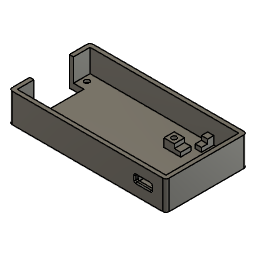
case_body (Autodesk Fusion 360 design; units mm, degrees)
Autodesk Fusion 360 part; units mm, degrees
sketch "Sketch1" plane through (0, 0, 0) normal (0, 1, 0) x (1, 0, 0)
  line L0 (0, 0) -> (75.7, 0)
  line L1 (75.7, 0) -> (75.7, -39.1)
  line L2 (75.7, -39.1) -> (0, -39.1)
  line L3 (0, 0) -> (0, -10)
  line L4 (0, -10) -> (7, -10)
  line L5 (7, -10) -> (7, -29.1)
  line L6 (7, -29.1) -> (0, -29.1)
  line L7 (0, -29.1) -> (0, -39.1)
  dimension "d1" = 75.7
  dimension "d2" = 39.1
  dimension "d67" = 10
  dimension "d68" = 10
  dimension "d69" = 7
  constraint horizontal L0
  constraint vertical L1
  constraint horizontal L2
  constraint coincident L0.start L3.start
  constraint vertical L3
  constraint perpendicular L3 L4
  constraint perpendicular L4 L5
  constraint perpendicular L3 L6
  constraint perpendicular L2 L7
  constraint collinear L3 L7
  measures "d1" distance of L0.start L0.end
  measures "d2" distance of L0.start L2.end
  measures "d67" distance of L0.start L3.end
  measures "d68" distance of L2.end L6.end
  measures "d69" distance of L5.end L6.end
extrude "Extrude1" add sketch "Sketch1" along normal blind 3 makes body 1
sketch "Sketch2" plane through (0, 3, 0) normal (0, 1, 0) x (-1, 0, 0)
  line L0 (-75.7, 0) -> (0, 0)
  line L1 (0, 0) -> (-75.7, 0)
  line L2 (-73.7, 2) -> (-2, 2)
  line L3 (-2, 2) -> (-2, 37.1)
  line L4 (-2, 37.1) -> (-73.7, 37.1)
  line L5 (-73.7, 37.1) -> (-73.7, 2)
  line L6 (0, 39.1) -> (-75.7, 39.1)
  line L7 (0, 0) -> (0, 39.1)
  line L8 (-75.7, 0) -> (-75.7, 39.1)
  line L9 (0, 0) -> (0, 10)
  line L10 (0, 10) -> (-7, 10)
  line L11 (-7, 10) -> (-7, 29.1)
  line L12 (-7, 29.1) -> (0, 29.1)
  line L13 (0, 29.1) -> (0, 39.1)
  point P0 (-75.7, 39.1)
  dimension "d31" = 2
  dimension "d34" = 2
  dimension "d35" = 2
  dimension "d36" = 2
  constraint horizontal L1
  constraint horizontal L2
  constraint coincident L0.end L1.start
  constraint vertical L3
  constraint horizontal L4
  constraint vertical L5
  constraint perpendicular L6 L7
  constraint perpendicular L6 L8
  constraint coincident P0 L6.end
  measures "d31" distance of L1 L2
  measures "d34" distance of L4 L6
  measures "d35" distance of L3 L7
  measures "d36" distance of L5 L8
extrude "Extrude2" add sketch "Sketch2" along normal blind 11 contours L0 L1 L2 L3 L4 L5 L6 L7 L8 L9 L10 L12 L13 bodies 1
sketch "Sketch3" plane through (0, 3, 0) normal (0, 1, 0) x (-1, 0, 0)
  line L0 (-73.7, 2) -> (-70.7, 2)
  line L1 (-70.7, 2) -> (-70.7, 5)
  line L2 (-70.7, 5) -> (-73.7, 5)
  line L3 (-73.7, 5) -> (-73.7, 2)
  line L4 (-55.6, 37.1) -> (-50.6, 37.1)
  line L5 (-50.6, 37.1) -> (-50.6, 32.1)
  line L6 (-50.6, 32.1) -> (-55.6, 32.1)
  line L7 (-55.6, 32.1) -> (-55.6, 37.1)
  line L8 (-58.7, 2) -> (-61.7, 2)
  line L9 (-61.7, 2) -> (-61.7, 5)
  line L10 (-61.7, 5) -> (-58.7, 5)
  line L11 (-58.7, 5) -> (-58.7, 2)
  line L12 (-50.6, 15) -> (-55.6, 15)
  line L13 (-55.6, 15) -> (-55.6, 10)
  line L14 (-50.6, 15) -> (-50.6, 10)
  line L15 (-50.6, 10) -> (-55.6, 10)
  line L16 (-73.7, 2) -> (-73.7, 37.1)
  line L17 (-2, 2) -> (-73.7, 2)
  line L18 (-73.7, 37.1) -> (-2, 37.1)
  dimension "d20" = 5
  dimension "d21" = 5
  dimension "d28" = 3
  dimension "d29" = 5
  dimension "d47" = 3
  dimension "d49" = 5
  dimension "d83" = 3
  dimension "d84" = 12
  dimension "d85" = 18.1
  dimension "d86" = 8
  constraint horizontal L0
  constraint vertical L1
  constraint vertical L3
  constraint horizontal L4
  constraint vertical L5
  constraint horizontal L6
  constraint vertical L7
  constraint horizontal L8
  constraint vertical L9
  constraint vertical L11
  constraint horizontal L12
  constraint vertical L13
  constraint collinear L2 L10
  constraint collinear L7 L13
  constraint perpendicular L9 L10
  constraint perpendicular L12 L14
  constraint coincident L8.start L17
  constraint coincident L0.end L17
  constraint coincident L2.end L16
  constraint coincident L4.end L18
  measures "d20" distance of L5.end L6.end
  measures "d21" distance of L4.end L5.end
  measures "d28" distance of L8.start L8.end
  measures "d29" distance of L12.start L12.end
  measures "d47" horizontal distance of L1.end L2.end
  measures "d49" distance of L12.start L14.end
  measures "d83" distance of L8.start L10.end
  measures "d84" distance of L9 L16
  measures "d85" distance of L7 L16
  measures "d86" distance of L15 L17
extrude "Extrude5" add sketch "Sketch3" along normal blind 4 separate body makes body 2 at (73.7, 4.3333, 4) makes body 3 at (58.7, 4.3333, 4) makes body 4 at (53.9333, 3, 35.4333) makes body 5 at (53.9333, 3, 11.6667)
sketch "Sketch5" plane through (0, 3, 0) normal (0, 1, 0) x (-1, 0, 0)
  line L0 (-70.7, 5) -> (-73.7, 5)
  line L1 (-73.7, 5) -> (-73.7, 8)
  line L2 (-73.7, 8) -> (-70.7, 8)
  line L3 (-70.7, 8) -> (-70.7, 5)
  line L4 (-55.6, 32.1) -> (-58.7, 32.1)
  line L5 (-58.7, 32.1) -> (-58.7, 37.1)
  line L6 (-58.7, 37.1) -> (-55.6, 37.1)
  line L7 (-55.6, 37.1) -> (-55.6, 32.1)
  line L8 (-73.7, 37.1) -> (-70.7, 37.1)
  line L9 (-70.7, 37.1) -> (-70.7, 32.1)
  line L10 (-70.7, 32.1) -> (-73.7, 32.1)
  line L11 (-73.7, 32.1) -> (-73.7, 37.1)
  line L12 (-58.7, 5) -> (-61.7, 5)
  line L13 (-61.7, 5) -> (-61.7, 8)
  line L14 (-61.7, 8) -> (-58.7, 8)
  line L15 (-58.7, 8) -> (-58.7, 5)
  line L16 (-58.7, 10) -> (-58.7, 15)
  line L17 (-58.7, 15) -> (-55.6, 15)
  line L18 (-55.6, 15) -> (-55.6, 10)
  line L19 (-55.6, 10) -> (-58.7, 10)
  line L20 (-2, 29.1) -> (-2, 37.1)
  line L21 (-2, 37.1) -> (-73.7, 37.1)
  line L22 (-73.7, 37.1) -> (-73.7, 2)
  line L23 (-73.7, 2) -> (-2, 2)
  line L24 (-2, 2) -> (-2, 10)
  line L25 (-2, 10) -> (-7, 10)
  line L26 (-7, 10) -> (-7, 29.1)
  line L27 (-7, 29.1) -> (-2, 29.1)
  point P0 (-73.7, 5)
  point P1 (-55.6, 37.1)
  point P2 (-58.7, 5)
  point P3 (-73.7, 37.1)
  point P4 (-55.6, 10)
  point P5 (-55.6, 15)
  point P6 (-61.7, 5)
  point P7 (-70.7, 5)
  point P8 (-55.6, 32.1)
  dimension "d43" = 3
  constraint horizontal L0
  constraint vertical L1
  constraint vertical L3
  constraint coincident P0 L0.end
  constraint horizontal L4
  constraint horizontal L6
  constraint vertical L7
  constraint coincident P1 L6.end
  constraint horizontal L8
  constraint vertical L9
  constraint horizontal L10
  constraint vertical L11
  constraint collinear L3 L9
  constraint collinear L4 L10
  constraint horizontal L12
  constraint vertical L13
  constraint horizontal L14
  constraint vertical L15
  constraint coincident P2 L12.start
  constraint collinear L2 L14
  constraint vertical L16
  constraint horizontal L17
  constraint vertical L18
  constraint collinear L15 L16
  constraint collinear L5 L16
  constraint coincident P3 L8.start
  constraint coincident P4 L18.end
  constraint perpendicular L16 L19
  constraint coincident P5 L17.end
  constraint coincident P6 L12.end
  constraint coincident P7 L0.start
  constraint coincident P8 L4.start
  measures "d43" distance of P2 L14.end
extrude "Extrude6" add sketch "Sketch5" along normal blind 2 contours L0 L1 L2 L3 L22 | L8 L9 L10 L11 L21 L22 | L4 L5 L6 L7 L21 | L12 L13 L14 L15 | L16 L17 L18 L19 bodies 1 3 5 2 4
hole "Hole6" at (53.1, 7, 12.5) direction (0, -1, 0) diameter 2.4 end up to surface (7 mm away) bodies 1
hole "Hole7" at (53.1, 7, 34.6) direction (0, -1, 0) diameter 2.4 end up to surface (7 mm away) bodies 1
sketch "Sketch7" plane through (0, 3, 0) normal (0, 1, 0) x (-1, 0, 0)
  line L0 (-58.7, 8) -> (-58.7, 2)
  line L1 (-58.7, 2) -> (-2, 2)
  line L2 (-2, 2) -> (-2, 10)
  line L3 (-2, 10) -> (-7, 10)
  line L4 (-7, 10) -> (-7, 29.1)
  line L5 (-7, 29.1) -> (-2, 29.1)
  line L6 (-2, 29.1) -> (-2, 37.1)
  line L7 (-2, 37.1) -> (-50.6, 37.1)
  line L8 (-50.6, 37.1) -> (-50.6, 32.1)
  line L9 (-50.6, 32.1) -> (-58.7, 32.1)
  line L10 (-58.7, 32.1) -> (-58.7, 37.1)
  line L11 (-58.7, 37.1) -> (-70.7, 37.1)
  line L12 (-70.7, 37.1) -> (-70.7, 32.1)
  line L13 (-70.7, 32.1) -> (-73.7, 32.1)
  line L14 (-73.7, 32.1) -> (-73.7, 8)
  line L15 (-73.7, 8) -> (-70.7, 8)
  line L16 (-70.7, 8) -> (-70.7, 2)
  line L17 (-70.7, 2) -> (-61.7, 2)
  line L18 (-61.7, 2) -> (-61.7, 8)
  line L19 (-61.7, 8) -> (-58.7, 8)
  line L20 (-50.6, 10) -> (-55.6, 10)
  line L21 (-55.6, 10) -> (-58.7, 10)
  line L22 (-58.7, 10) -> (-58.7, 15)
  line L23 (-58.7, 15) -> (-50.6, 15)
  line L24 (-50.6, 15) -> (-50.6, 10)
  point P0 (-4.5, 6)
  point P1 (-4.5, 33.1)
  dimension "d96" = 2.5
  dimension "d97" = 2
  dimension "d98" = 4
  dimension "d99" = 4
  dimension "d100" = 4
  dimension "d101" = 2.5
  measures "d96" distance of L2 P0
  measures "d98" distance of L3 P0
  measures "d99" distance of L1 P0
  measures "d100" distance of L5 P1
  measures "d101" distance of L4 P1
hole "Hole9" at (4.5, 3, 6) at (4.5, 3, 33.1) direction (0, -1, 0) diameter 2.4 end up to surface (3 mm away) bodies 1
sketch "Sketch8" plane through (0, 0, 0) normal (0, -1, 0) x (1, 0, 0)
  circle A0 centre (4.5, 6) radius 1.2
  circle A1 centre (4.5, 33.1) radius 1.2
  circle A2 centre (53.1, 34.6) radius 1.2
  circle A3 centre (53.1, 12.5) radius 1.2
  line L0 (0, 10) -> (0, 0)
  line L1 (0, 0) -> (75.7, 0)
  line L2 (75.7, 0) -> (75.7, 39.1)
  line L3 (75.7, 39.1) -> (0, 39.1)
  line L4 (0, 39.1) -> (0, 29.1)
  line L5 (0, 29.1) -> (7, 29.1)
  line L6 (7, 29.1) -> (7, 10)
  line L7 (7, 10) -> (0, 10)
  line L8 (6.8, 34.4279) -> (4.5, 35.7558)
  line L9 (4.5, 35.7558) -> (2.2, 34.4279)
  line L10 (2.2, 34.4279) -> (2.2, 31.7721)
  line L11 (2.2, 31.7721) -> (4.5, 30.4442)
  line L12 (4.5, 30.4442) -> (6.8, 31.7721)
  line L13 (6.8, 31.7721) -> (6.8, 34.4279)
  line L14 (6.8, 7.3279) -> (4.5, 8.6558)
  line L15 (4.5, 8.6558) -> (2.2, 7.3279)
  line L16 (2.2, 7.3279) -> (2.2, 4.6721)
  line L17 (2.2, 4.6721) -> (4.5, 3.3442)
  line L18 (4.5, 3.3442) -> (6.8, 4.6721)
  line L19 (6.8, 4.6721) -> (6.8, 7.3279)
  line L20 (55.4, 35.9279) -> (53.1, 37.2558)
  line L21 (53.1, 37.2558) -> (50.8, 35.9279)
  line L22 (50.8, 35.9279) -> (50.8, 33.2721)
  line L23 (50.8, 33.2721) -> (53.1, 31.9442)
  line L24 (53.1, 31.9442) -> (55.4, 33.2721)
  line L25 (55.4, 33.2721) -> (55.4, 35.9279)
  line L26 (55.4, 13.8279) -> (53.1, 15.1558)
  line L27 (53.1, 15.1558) -> (50.8, 13.8279)
  line L28 (50.8, 13.8279) -> (50.8, 11.1721)
  line L29 (50.8, 11.1721) -> (53.1, 9.8442)
  line L30 (53.1, 9.8442) -> (55.4, 11.1721)
  line L31 (55.4, 11.1721) -> (55.4, 13.8279)
  point P0 (4.5, 33.1)
  point P1 (4.5, 6)
  point P2 (53.1, 34.6)
  point P3 (53.1, 12.5)
  dimension "d105" = 4.6
  dimension "d106" = 4.6
  dimension "d107" = 4.6
  dimension "d108" = 4.6
  constraint coincident P0 A1.centre
  constraint coincident A0.centre P1
  constraint coincident P2 A2.centre
  constraint coincident P3 A3.centre
  measures "d105" distance of L10 L13
  measures "d106" distance of L16 L19
  measures "d107" distance of L22 L25
  measures "d108" distance of L28 L31
extrude "Extrude8" cut sketch "Sketch8" against normal blind 1.8 contours L8 L9 L10 L11 L12 L13 | L14 L15 L16 L17 L18 L19 | L20 L21 L22 L23 L24 L25 | L26 L27 L28 L29 L30 L31 bodies 1
sketch "Sketch6" plane through (0, 0, 39.1) normal (0, 0, 1) x (1, 0, 0)
  line L0 (0, 0) -> (75.7, 0)
  line L1 (75.7, 0) -> (75.7, 14)
  line L2 (75.7, 14) -> (0, 14)
  line L3 (0, 14) -> (0, 0)
  line L4 (61.2, 8.7) -> (68.2, 8.7)
  line L5 (68.7, 8.2) -> (68.7, 6.2)
  line L6 (68.2, 5.7) -> (61.2, 5.7)
  line L7 (60.7, 6.2) -> (60.7, 8.2)
  arc A0 (61.2, 8.7) -> (60.7, 8.2) centre (61.2, 8.2) ccw
  arc A1 (60.7, 6.2) -> (61.2, 5.7) centre (61.2, 6.2) ccw
  arc A2 (68.2, 5.7) -> (68.7, 6.2) centre (68.2, 6.2) ccw
  arc A3 (68.7, 8.2) -> (68.2, 8.7) centre (68.2, 8.2) ccw
  point P0 (60.7, 8.7)
  point P1 (68.7, 8.7)
  point P2 (60.7, 5.7)
  dimension "d73" = 7
  dimension "d75" = 3
  dimension "d76" = 8
  dimension "d80" = 0.5
  dimension "d111" = 5.3
  constraint horizontal L4
  constraint vertical L5
  constraint horizontal L6
  constraint vertical L7
  constraint coincident P0 L7
  constraint coincident P0 L4
  constraint tangent L7 A0
  constraint tangent L4 A0
  constraint coincident P2 L7
  constraint coincident P2 L6
  constraint tangent L7 A1
  constraint tangent L6 A1
  constraint equal A0 A1
  constraint tangent L6 A2
  constraint tangent L5 A2
  constraint equal A0 A2
  constraint coincident P1 L4
  constraint coincident P1 L5
  constraint tangent L4 A3
  constraint tangent L5 A3
  constraint equal A0 A3
  measures "d73" distance of L1 L5
  measures "d75" distance of P0 P2
  measures "d76" distance of P0 P1
  measures "d80" radius of A0
  measures "d111" distance of L2 L4
extrude "Extrude7" cut sketch "Sketch6" against normal up to surface (2 mm away) contours L4 L5 L6 L7 A0 A1 A2 A3 bodies 1
fillet "Fillet2" radius 0.5 16 edges at (60.7, 7.2, 39.1) (60.8464, 8.5536, 39.1) (64.7, 8.7, 39.1) (68.5536, 8.5536, 39.1) (68.7, 7.2, 39.1) (68.5536, 5.8464, 39.1) (64.7, 5.7, 39.1) (60.8464, 5.8464, 39.1) (68.7, 7.2, 37.1) (68.5536, 8.5536, 37.1) (64.7, 8.7, 37.1) (60.8464, 8.5536, 37.1) (60.7, 7.2, 37.1) (60.8464, 5.8464, 37.1) (64.7, 5.7, 37.1) (68.5536, 5.8464, 37.1) on bodies 1
fillet "Fillet3" radius 1.5 4 edges at (75.7, 7, 39.1) (75.7, 7, 0) (0, 7, 39.1) (0, 7, 0) on bodies 1
